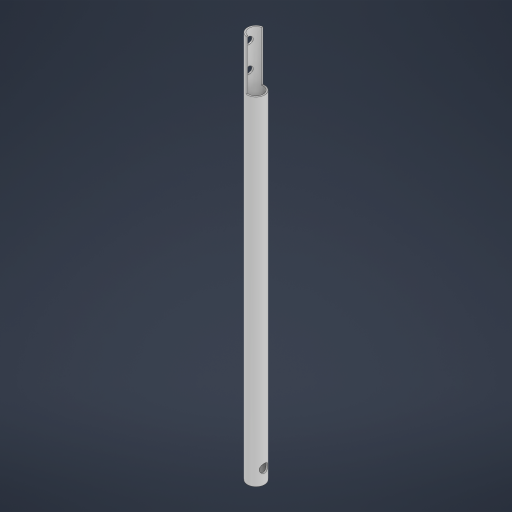
# Autodesk Inventor part: pipe
Saved by Autodesk Inventor 2023 (Build 270158000, 158)
## iProperties
Created: 2022-04-24
Part Number: pipe
Material: Aluminum 6061
Document SubType Name: Modeling
Designer: Norbert Ligas
Density: 2.7 g/cm^3
Appearance: Aluminum - Polished
pipe_length: 271,147 mm
connector_min_length: 306,147 mm
bar_connection: 35,000 mm
Author: Norbert Ligas
Autodesk Inventor part; units mm, degrees
ref_plane "XZ Plane" through (0, 0, 0) normal (0, 1, 0) x (-1, 0, 0)
ref_plane "XY Plane" through (0, 0, 0) normal (0, 0, 1) x (1, 0, 0)
sketch "Sketch1" plane through (0, 0, 0) normal (0, 1, 0) x (-1, 0, 0)
  circle A0 centre (0, 0) radius 5
  circle A1 centre (0, 0) radius 6
  dimension "d0" = 12
  dimension "d1" = 1
  constraints: 2 centre point, 2 coincident
  measures "d0" diameter of A1
  measures "d1" radial gap between concentric circles of A0 A1
extrude "Extrusion1" add sketch "Sketch1" along normal blind 271.1467
ref_plane "Work Plane3" through (6, 0, 0) normal (1, 0, 0) x (0, 1, 0)
sketch "Sketch2" plane through (6, 0, 0) normal (1, 0, 0) x (0, 1, 0)
  line L0 (0, -6) -> (271.1467, -6) projected
  line L1 (0, 6) -> (271.1467, 6) projected
  line L2 (271.1467, -6) -> (271.1467, 6) projected
  line L3 (-104.525, 0) -> (627.1502, 0) projected
  point P0 (0, 0)
  point P1 (10, 0)
  point P2 (271.1467, 0)
  dimension "d20" = 10
  constraints: 1 midpoint, 1 point on line
  measures "d20" distance of point (0, 0) point (10, 0)
hole "Hole1" at (6, 10, 0) direction (-1, 0, 0) diameter 6 end up to face face through (0, 0, 0) facing (0, 1, 0) round with radius 5 far side no
sketch "Sketch3" plane through (6, 0, 0) normal (1, 0, 0) x (0, 1, 0)
  line L0 (-54.2293, 0) -> (325.3761, 0) projected
  line L1 (271.1467, -6) -> (271.1467, 6) projected
  line L2 (236.1467, 6) -> (271.1467, 6)
  line L3 (271.1467, 6) -> (271.1467, -6)
  line L4 (271.1467, -6) -> (236.1467, -6)
  line L5 (236.1467, -6) -> (236.1467, 6)
  point P0 (0, 0)
  point P1 (245.6467, 0)
  point P2 (263.6467, 0)
  dimension "d22" = 7.5
  dimension "d23" = 18
  dimension "d24" = 35
  constraints: 8 end point, 2 parallel, 2 point on line, 1 horizontal, 1 perpendicular
  measures "d22" distance from line of L1 point (263.647, 0)
  measures "d23" distance of point (245.647, 0) point (263.647, 0)
  measures "d24" distance between parallel lines of L1 L5
extrude "Extrusion2" cut sketch "Sketch3" against normal blind 7
hole "Hole3" at (6, 263.6467, 0) at (6, 245.6467, 0) direction (-1, 0, 0) diameter 5 end through all
equation "\"d2\" = pipe_length"
equation "\"d24\" = bar_connection"
equation "\"d25\" = pipe_cutout"
equation "\"pipe_length\" = connector_min_length - bar_connection"
equation "\"alfa\" = 45deg"
equation "\"bar_connection\" = 35"
equation "\"pipe_cutout\" = 7"
equation "\"connector_min_length\" = 306.146746"
body "Solid1"
